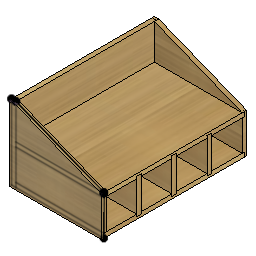
fusion_360_shelf (Autodesk Fusion 360 design; units mm, degrees)
Autodesk Fusion 360 part; units mm, degrees
note: some values were not read from the file. Set by a fixed rule: which sketch regions a step uses.
sketch "Bottom" plane through (0, 0, 0) normal (0, 0, 1) x (1, 0, 0)
  line L0 (0, 0) -> (260.35, 0)
  line L1 (260.35, 0) -> (260.35, 406.4)
  line L2 (260.35, 406.4) -> (0, 406.4)
  line L3 (0, 406.4) -> (0, 0)
  dimension "d10" = 260.35
  dimension "d11" = 406.4
  constraint horizontal L0
  constraint vertical L1
  constraint horizontal L2
  constraint vertical L3
  constraint coincident L0.start L3.end
  measures "d10" distance of L0.start L0.end
  measures "d11" distance of L0.start L2.end
extrude "raise_bottom" add sketch "Bottom" along normal blind 12.7 makes body 1
sketch "draw_slot_dado" plane through (0, 0, 12.7) normal (0, 0, 1) x (-1, 0, 0)
  line L0 (0, -406.4) -> (0, 0)
  line L1 (0, 0) -> (-260.35, 0)
  line L2 (-260.35, 0) -> (-260.35, -406.4)
  line L3 (-260.35, -406.4) -> (0, -406.4)
  line L4 (0, -95.25) -> (-260.35, -95.25)
  line L5 (-260.35, -107.95) -> (0, -107.95)
  dimension "d40" = 95.25
  dimension "d41" = 12.7
  constraint coincident L0 L4.start
  constraint coincident L2 L4.end
  constraint perpendicular L2 L4
  constraint coincident L2 L5.start
  constraint coincident L0 L5.end
  constraint perpendicular L0 L5
  measures "d40" distance of L1 L4
  measures "d41" distance of L4 L5
extrude "cut_slot_dado" cut sketch "draw_slot_dado" against normal blind 6.35 contours L0 L2 L4 L5 bodies 1
pattern_linear "cut_remaining_slots" count 3 spacing 101.6 along (0, 1, 0) of "cut_slot_dado"
copy_body "CopyPasteBodies4" bodies 1 makes body 2
move_body "move_top_up" bodies 2 to x (1, 0, 0) y (0, 1, 0) z (0, 0, 1) at (0, 0, 101.6)
sketch "drop_top_left_center" plane through (0, 0, 0) normal (0, -1, 0) x (1, 0, 0)
  line L0 (0, 101.6) -> (260.35, 101.6)
  line L1 (260.35, 101.6) -> (260.35, 114.3)
  line L2 (260.35, 114.3) -> (0, 114.3)
  line L3 (0, 114.3) -> (0, 101.6)
  line L4 (130.175, 114.3) -> (130.175, 101.6) construction
  line L5 (0, 107.95) -> (260.35, 107.95) construction
  point P0 (130.175, 114.3)
  point P1 (130.175, 101.6)
  point P2 (0, 107.95)
  point P3 (260.35, 107.95)
  point P4 (130.175, 107.95)
  constraint midpoint L2 P0
  constraint midpoint L0 P1
  constraint midpoint L3 P2
  constraint midpoint L1 P3
  constraint coincident P0 L4.start
  constraint coincident P1 L4.end
  constraint coincident P2 L5.start
  constraint coincident P3 L5.end
  constraint midpoint L5 P4
sketch "draw_top_right_center (1)" plane through (0, 406.4, 0) normal (0, 1, 0) x (-1, 0, 0)
  line L0 (-260.35, 101.6) -> (0, 101.6)
  line L1 (0, 101.6) -> (0, 114.3)
  line L2 (0, 114.3) -> (-260.35, 114.3)
  line L3 (-260.35, 114.3) -> (-260.35, 101.6)
  line L4 (-130.175, 114.3) -> (-130.175, 101.6) construction
  line L5 (-260.35, 107.95) -> (0, 107.95) construction
  point P0 (-130.175, 107.95)
  constraint midpoint L2 L4.start
  constraint midpoint L0 L4.end
  constraint midpoint L3 L5.start
  constraint midpoint L1 L5.end
  constraint midpoint L5 P0
sketch "draw_top_rotation_axis" plane through (0, 406.4, 0) normal (0, 1, 0) x (-1, 0, 0)
  line L0 (-130.175, 107.95, -406.4) -> (-130.175, 107.95, 0)
  point P0 (-130.175, 107.95)
  point P1 (-130.175, 107.95)
  constraint coincident P0 P1
  constraint coincident P1 P0
move_body "rotate_top_180" bodies 2 to x (-1, 0, 0) y (0, 1, 0) z (0, 0, -1) at (260.35, 0, 215.9)
sketch "inner_slot" plane through (260.35, 0, 0) normal (1, 0, 0) x (0, 1, 0)
  line L0 (298.45, 12.7) -> (209.55, 12.7)
  line L1 (209.55, 12.7) -> (209.55, 6.35)
  line L2 (209.55, 6.35) -> (196.85, 6.35)
  line L3 (196.85, 6.35) -> (196.85, 12.7)
  line L4 (196.85, 12.7) -> (107.95, 12.7)
  line L5 (107.95, 12.7) -> (107.95, 6.35)
  line L6 (107.95, 6.35) -> (95.25, 6.35)
  line L7 (95.25, 6.35) -> (95.25, 12.7)
  line L8 (95.25, 12.7) -> (0, 12.7)
  line L9 (0, 12.7) -> (0, 0)
  line L10 (0, 0) -> (406.4, 0)
  line L11 (406.4, 0) -> (406.4, 12.7)
  line L12 (95.25, 6.35) -> (107.95, 6.35)
  line L13 (107.95, 6.35) -> (107.95, 107.95)
  line L14 (107.95, 107.95) -> (95.25, 107.95)
  line L15 (95.25, 107.95) -> (95.25, 6.35)
  line L16 (311.15, 12.7) -> (311.15, 6.35)
  line L17 (311.15, 6.35) -> (298.45, 6.35)
  line L18 (298.45, 6.35) -> (298.45, 12.7)
  line L19 (406.4, 12.7) -> (311.15, 12.7)
  point P0 (107.95, 107.95)
  constraint horizontal L12
  constraint vertical L13
  constraint horizontal L14
  constraint vertical L15
  constraint coincident P0 L13.end
  constraint coincident L6.end L7.start
extrude "Extrude15" add sketch "inner_slot" against normal blind 260.35 separate body contours L5 L6 L7 L12 L13 L14 L15 makes body 3
copy_body "Body->Comp1" bodies 3 removing the originals makes body 4 in component "inner_slot"
pattern_linear "R-Pattern1" count 3 spacing 101.6 along (0, 1, 0) of bodies 4 makes body 5 at (173.5667, 196.85, 76.2) makes body 6 at (173.5667, 298.45, 76.2) in component "inner_slot"
sketch "back" plane through (0, 0, 0) normal (-1, 0, 0) x (0, -1, 0)
  line L0 (-311.15, 12.7) -> (-406.4, 12.7)
  line L1 (-406.4, 12.7) -> (-406.4, 0)
  line L2 (-406.4, 0) -> (0, 0)
  line L3 (0, 0) -> (0, 12.7)
  line L4 (0, 12.7) -> (-95.25, 12.7)
  line L5 (-95.25, 12.7) -> (-95.25, 6.35)
  line L6 (-95.25, 6.35) -> (-107.95, 6.35)
  line L7 (-107.95, 6.35) -> (-107.95, 12.7)
  line L8 (-107.95, 12.7) -> (-196.85, 12.7)
  line L9 (-196.85, 12.7) -> (-196.85, 6.35)
  line L10 (-196.85, 6.35) -> (-209.55, 6.35)
  line L11 (-209.55, 6.35) -> (-209.55, 12.7)
  line L12 (-406.4, 0) -> (0, 0)
  line L13 (0, 0) -> (0, 215.9)
  line L14 (0, 215.9) -> (-406.4, 215.9)
  line L15 (-406.4, 215.9) -> (-406.4, 0)
  line L16 (-196.85, 101.6) -> (-196.85, 107.95)
  line L17 (-209.55, 107.95) -> (-209.55, 101.6)
  line L18 (-196.85, 107.95) -> (-209.55, 107.95)
  line L19 (-196.85, 101.6) -> (-107.95, 101.6)
  line L20 (-95.25, 101.6) -> (-95.25, 107.95)
  line L21 (-107.95, 107.95) -> (-107.95, 101.6)
  line L22 (-95.25, 107.95) -> (-107.95, 107.95)
  line L23 (-95.25, 101.6) -> (0, 101.6)
  line L24 (-406.4, 114.3) -> (-406.4, 101.6)
  line L25 (0, 114.3) -> (0, 101.6)
  line L26 (-406.4, 114.3) -> (0, 114.3)
  line L27 (-209.55, 12.7) -> (-209.55, 6.35)
  line L28 (-209.55, 6.35) -> (-196.85, 6.35)
  line L29 (-196.85, 6.35) -> (-196.85, 12.7)
  line L30 (-107.95, 12.7) -> (-196.85, 12.7)
  line L31 (-107.95, 12.7) -> (-107.95, 6.35)
  line L32 (-107.95, 6.35) -> (-95.25, 6.35)
  line L33 (-95.25, 6.35) -> (-95.25, 12.7)
  line L34 (0, 12.7) -> (-95.25, 12.7)
  line L35 (0, 0) -> (0, 12.7)
  line L36 (0, 0) -> (-406.4, 0)
  line L37 (-406.4, 0) -> (-406.4, 12.7)
  line L38 (-107.95, 107.95) -> (-95.25, 107.95)
  line L39 (-95.25, 107.95) -> (-95.25, 6.35)
  line L40 (-95.25, 6.35) -> (-107.95, 6.35)
  line L41 (-107.95, 6.35) -> (-107.95, 107.95)
  line L42 (-209.55, 12.7) -> (-298.45, 12.7)
  line L43 (-298.45, 12.7) -> (-298.45, 6.35)
  line L44 (-298.45, 6.35) -> (-311.15, 6.35)
  line L45 (-311.15, 6.35) -> (-311.15, 12.7)
  line L46 (-298.45, 101.6) -> (-298.45, 107.95)
  line L47 (-311.15, 107.95) -> (-311.15, 101.6)
  line L48 (-298.45, 107.95) -> (-311.15, 107.95)
  line L49 (-298.45, 101.6) -> (-209.55, 101.6)
  line L50 (-311.15, 12.7) -> (-311.15, 6.35)
  line L51 (-311.15, 6.35) -> (-298.45, 6.35)
  line L52 (-298.45, 6.35) -> (-298.45, 12.7)
  line L53 (-209.55, 12.7) -> (-298.45, 12.7)
  line L54 (-406.4, 101.6) -> (-311.15, 101.6)
  line L55 (-311.15, 12.7) -> (-406.4, 12.7)
  dimension "d115" = 406.4
  dimension "d116" = 215.9
  constraint horizontal L12
  constraint vertical L13
  constraint horizontal L14
  constraint vertical L15
  constraint coincident L1.end L2.start
  constraint horizontal L38
  constraint vertical L39
  constraint horizontal L40
  constraint vertical L41
  constraint coincident L5.end L6.start
  constraint coincident L21.start L22.end
  measures "d115" distance of L1.end L2.end
  measures "d116" distance of L1.end L14.end
extrude "Extrude16" add sketch "back" against normal blind 6.35 separate body makes body 7
extrude "Extrude17" add 1 faces at (0, 135.4667, 148.1667) along direction (-1, 0, 0) blind 6.35 on bodies 7 bodies 7
extrude "Extrude19" cut sketch "back" against normal blind 6.35 contours L5 L6 L7 L20 L21 L22 L31 L32 L33 L38 L39 L40 L41 bodies 7
pattern_linear "R-Pattern7" count 3 spacing 101.6 along (0, 1, 0) of "Extrude19"
extrude "Extrude20" cut sketch "back" against normal blind 6.35 contours L0 L1 L2 L3 L4 L5 L6 L7 L8 L9 L10 L11 L12 L13 L15 L27 L28 L29 L30 L31 L32 L33 L34 L35 L36 L37 L39 L40 L41 L42 L43 L44 L45 L50 L51 L52 L53 L55 | L13 L15 L16 L17 L18 L19 L20 L21 L22 L23 L24 L25 L26 L38 L39 L41 L46 L47 L48 L49 L54 bodies 7
sketch "left_side" plane through (0, 0, 0) normal (0, -1, 0) x (1, 0, 0)
  line L0 (0, 0) -> (260.35, 0)
  line L1 (260.35, 0) -> (260.35, 12.7)
  line L2 (260.35, 12.7) -> (0, 12.7)
  line L3 (0, 12.7) -> (0, 0)
  line L4 (260.35, 0) -> (-6.35, 0)
  line L5 (-6.35, 0) -> (-6.35, 215.9)
  line L6 (6.35, 215.9) -> (260.35, 114.3)
  line L7 (260.35, 114.3) -> (260.35, 0)
  line L8 (6.35, 215.9) -> (-6.35, 215.9)
  line L9 (6.35, 215.9) -> (6.35, 0)
  line L10 (260.35, 12.7) -> (6.35, 12.7)
  line L11 (6.35, 101.6) -> (260.35, 101.6)
  line L12 (260.35, 114.3) -> (6.35, 114.3)
  point P0 (-6.35, 215.9)
  point P1 (6.35, 215.9)
  point P2 (260.35, 114.3)
  dimension "d131" = 12.7
  dimension "d132" = 279.4
  dimension "d133" = 12.7
  dimension "d134" = 88.9
  constraint horizontal L4
  constraint vertical L5
  constraint coincident P0 L5.end
  constraint coincident L0.end L1.start
  constraint coincident P1 L6.start
  constraint coincident P2 L6.end
  constraint coincident L4 L9.end
  constraint coincident L7 L1.end
  constraint coincident L9 L10.end
  constraint perpendicular L9 L10
  constraint coincident L9 L11.start
  constraint coincident L7 L11.end
  constraint perpendicular L7 L11
  constraint coincident L9 L12.end
  constraint perpendicular L9 L12
  measures "d131" distance of L5 L9
  measures "d133" distance of L4 L10
  measures "d134" distance of L10 L11
extrude "Extrude21" add sketch "left_side" along normal blind 6.35 separate body makes body 8
extrude "Extrude22" add sketch "left_side" against normal blind 6.35 contours L2 L7 L9 L10 L11 | L6 L9 L12 bodies 8
mirror "Mirror2" about plane through (0, 6.35, 0) normal (0, 1, 0) of bodies 8 makes body 9
move_body "Move9" bodies 9 to x (1, 0, 0) y (0, 1, 0) z (0, 0, 1) at (0, 393.7, 0)
component "inner_slot" placed x (1, 0, 0) y (0, 1, 0) z (0, 0, 1) at (0, 0, 0)
equation "plywoodThickness = 0.5 in"
equation "InnerSlotWidth = 3.5 in"
equation "InnerSlotHeight = 3.5 in"
equation "InnerSlotDepth = 10 in"
equation "dadoDepth = plywoodThickness / 2"
equation "bottomWidth = ( InnerSlotWidth + plywoodThickness ) * numberOfSlots"
equation "bottomDepth = InnerSlotDepth + dadoDepth"
equation "d10 = bottomDepth"
equation "d11 = bottomWidth"
equation "numberOfSlots = 4"
equation "d38 = plywoodThickness"
equation "d40 = InnerSlotWidth + dadoDepth"
equation "d41 = plywoodThickness"
equation "d42 = -dadoDepth"
equation "d44 = numberOfSlots - 1"
equation "d46 = InnerSlotWidth + plywoodThickness"
equation "d50 = InnerSlotHeight + plywoodThickness"
equation "topShelfHeight = 4 in"
equation "BackHeight = topShelfHeight + InnerSlotHeight + ( plywoodThickness * 2 )"
equation "d103 = -bottomDepth"
equation "d111 = numberOfSlots - 1"
equation "d113 = InnerSlotWidth + plywoodThickness"
equation "d115 = bottomWidth"
equation "d116 = BackHeight"
equation "d117 = -dadoDepth"
equation "d119 = dadoDepth"
equation "d123 = -dadoDepth"
equation "d125 = numberOfSlots - 1"
equation "d127 = -InnerSlotWidth - plywoodThickness"
equation "d129 = -dadoDepth"
equation "d131 = plywoodThickness"
equation "d133 = plywoodThickness"
equation "d134 = InnerSlotHeight"
equation "d135 = dadoDepth"
equation "d137 = -dadoDepth"
equation "d142 = bottomWidth - plywoodThickness"
named bodies: "Bottom", "Top", "inner_slot", "inner_slot (1)", "Back", "Left_Side", "Right_Side", "inner_slot (2)"
